Autodesk Fusion 360 part; units mm, degrees
(part 2 of 5)
sketch "Base" plane through (0, 0, 0) normal (0, 1, 0) x (1, 0, 0) in component "GM67 + printer"
  line L0 (0, 0) -> (183.0748, 0)
  line L1 (196.0652, -7.5) -> (240.6025, -84.641)
  line L2 (235.1122, -105.1314) -> (174.4904, -140.1314)
  line L3 (154, -134.641) -> (138.3301, -107.5)
  line L4 (125.3397, -100) -> (19, -100)
  line L5 (4, -115) -> (4, -142)
  line L6 (1, -145) -> (0, -145)
  line L7 (0, -145) -> (0, 0)
  arc A0 (196.0652, -7.5) -> (183.0748, 0) centre (183.0748, -15) ccw
  arc A1 (235.1122, -105.1314) -> (240.6025, -84.641) centre (227.6122, -92.141) ccw
  arc A2 (154, -134.641) -> (174.4904, -140.1314) centre (166.9904, -127.141) ccw
  arc A3 (138.3301, -107.5) -> (125.3397, -100) centre (125.3397, -115) ccw
  arc A4 (19, -100) -> (4, -115) centre (19, -115) ccw
  line L8 (4, -4) -> (183.0748, -4)
  arc A5 (192.6011, -9.5) -> (183.0748, -4) centre (183.0748, -15) ccw
  line L9 (192.6011, -9.5) -> (237.1384, -86.641)
  arc A6 (233.1122, -101.6673) -> (237.1384, -86.641) centre (227.6122, -92.141) ccw
  line L10 (233.1122, -101.6673) -> (172.4904, -136.6673)
  arc A7 (157.4641, -132.641) -> (172.4904, -136.6673) centre (166.9904, -127.141) ccw
  line L11 (157.4641, -132.641) -> (141.7942, -105.5)
  arc A8 (141.7942, -105.5) -> (125.3397, -96) centre (125.3397, -115) ccw
  line L12 (125.3397, -96) -> (19, -96)
  arc A9 (19, -96) -> (4, -103.3381) centre (19, -115) ccw
  line L13 (4, -103.3381) -> (4, -4)
  arc A10 (1, -145) -> (4, -142) centre (1, -142) ccw
  arc A11 (4, -12) -> (12, -4) centre (4, -4) ccw
  line L14 (4, -4) -> (9.6569, -9.6569) construction
  circle A12 centre (6.8284, -6.8284) radius 2
  line L15 (166.9904, -127.141) -> (161.5, -147.6314) construction
  spline S0 degree 2 poles (157.4641, -132.641) (166.9904, -127.141) (172.4904, -136.6673) knots 0 0 0 1.944544 1.944544 1.944544 weights 1 3 1
  circle A13 centre (165.1786, -133.9025) radius 2
  line L16 (192.6011, -9.5) -> (189.4806, -11.3016)
  line L17 (179.9994, -4) -> (179.9994, -6.8969)
  line L18 (181.9766, -9.7171) -> (186.9578, -11.5237)
  arc A14 (179.9994, -6.8969) -> (181.9766, -9.7171) centre (182.9994, -6.8969) ccw
  arc A15 (186.9578, -11.5237) -> (189.4806, -11.3016) centre (187.9806, -8.7035) ccw
  spline S1 degree 2 poles (233.1122, -101.6673) (227.6122, -92.141) (237.1384, -86.641) knots 0 0 0 1.944544 1.944544 1.944544 weights 1 3 1
  line L19 (227.6122, -92.141) -> (248.1025, -97.6314) construction
  circle A16 centre (234.3736, -93.9527) radius 2
  line L20 (179.9994, -4) -> (192.6011, -9.5) construction
  arc A17 (125.3397, -96) -> (109.3397, -96) centre (117.3397, -96) ccw
  line L21 (117.3397, -96) -> (117.3397, -88) construction
  circle A18 centre (117.3397, -93.1716) radius 2
  line L22 (4, -115) -> (0, -115)
  line L23 (186.3002, -6.75) -> (184.4672, -10.6204) construction
  circle A19 centre (185.872, -7.6542) radius 2
  circle A20 centre (6.8284, -6.8284) radius 2.25
  circle A21 centre (185.872, -7.6542) radius 2.25
  circle A22 centre (234.3736, -93.9527) radius 2.25
  circle A23 centre (117.3397, -93.1716) radius 2.25
  circle A24 centre (165.1786, -133.9025) radius 2.25
  line L24 (4, -53.669) -> (218.1021, -53.669) construction
  line L25 (135, -17.169) -> (72, -17.169)
  line L26 (72, -17.169) -> (72, -80.169)
  line L27 (72, -80.169) -> (135, -80.169)
  line L28 (135, -80.169) -> (135, -17.169)
  line L29 (135, -17.169) -> (72, -80.169) construction
  line L30 (72, -17.169) -> (135, -80.169) construction
  line L31 (133, -19.169) -> (74, -19.169)
  line L32 (74, -19.169) -> (74, -78.169) construction
  line L33 (74, -78.169) -> (133, -78.169) construction
  line L34 (133, -78.169) -> (133, -19.169) construction
  line L35 (133, -19.169) -> (74, -78.169) construction
  line L36 (74, -19.169) -> (133, -78.169) construction
  circle A25 centre (74, -78.169) radius 0.95
  circle A26 centre (74, -78.169) radius 3.45
  circle A27 centre (133, -78.169) radius 0.95
  circle A28 centre (133, -78.169) radius 3.45
  circle A29 centre (133, -19.169) radius 0.95
  circle A30 centre (133, -19.169) radius 3.45
  circle A31 centre (74, -19.169) radius 3.45
  circle A32 centre (74, -19.169) radius 0.95
  line L37 (49.5, -96) -> (49.5, -4)
  line L38 (53.5, -96) -> (53.5, -4)
  line L39 (53.5, -96) -> (53.5, -100)
  line L40 (53.5, -4) -> (53.5, 0)
  arc A33 (61.5, -96) -> (53.5, -88) centre (53.5, -96) ccw
  line L41 (53.5, -96) -> (59.1569, -90.3431) construction
  circle A34 centre (56.3284, -93.1716) radius 2
  circle A35 centre (56.3284, -93.1716) radius 2.25
  arc A36 (53.5, -12) -> (61.5, -4) centre (53.5, -4) ccw
  line L42 (53.5, -4) -> (59.1569, -9.6569) construction
  circle A37 centre (56.3284, -6.8284) radius 2
  circle A38 centre (56.3284, -6.8284) radius 2.25
  line L43 (49.5, -96) -> (4, -96)
  arc A39 (12, -96) -> (4, -88) centre (4, -96) ccw
  line L44 (4, -96) -> (9.6569, -90.3431) construction
  circle A40 centre (6.8284, -93.1716) radius 2
  circle A41 centre (6.8284, -93.1716) radius 2.25
  line L45 (117.3397, -96) -> (117.3397, -4) construction
  arc A42 (109.3397, -4) -> (125.3397, -4) centre (117.3397, -4) ccw
  line L46 (117.3397, -12) -> (117.3397, -4) construction
  line L47 (56.3284, -6.8284) -> (117.3397, -6.8284) construction
  circle A43 centre (117.3397, -6.8284) radius 2
  line L48 (56.3284, -93.1716) -> (117.3397, -93.1716) construction
  circle A44 centre (117.3397, -6.8284) radius 2.25
  line L49 (47.5, -96) -> (47.5, -95)
  line L50 (47.5, -95) -> (47.5, -4) construction
  line L51 (47.5, -12) -> (49.5, -12)
  arc A45 (47.5, -88) -> (39.5, -96) centre (47.5, -96) ccw
  line L52 (47.5, -88) -> (49.5, -88)
  line L53 (47.5, -96) -> (41.8431, -90.3431) construction
  circle A46 centre (44.6716, -93.1716) radius 2
  circle A47 centre (44.6716, -93.1716) radius 2.25
  arc A48 (39.5, -4) -> (47.5, -12) centre (47.5, -4) ccw
  line L54 (47.5, -4) -> (41.8431, -9.6569) construction
  circle A49 centre (44.6716, -6.8284) radius 2
  circle A50 centre (44.6716, -6.8284) radius 2.25
  line L55 (203.6221, -48.669) -> (205, -52.2911)
  line L56 (205, -52.2911) -> (204.352, -52.2911)
  line L57 (204.352, -52.2911) -> (203.5744, -50.122)
  spline S2 degree 2 poles (203.5744, -50.122) (203.4482, -49.7707) (203.3424, -49.3921) knots 0 0 0 1 1 1
  spline S3 degree 2 poles (203.3424, -49.3921) (203.2606, -49.6786) (203.1139, -50.0811) knots 0 0 0 1 1 1
  line L58 (203.1139, -50.0811) -> (202.309, -52.2911)
  line L59 (202.309, -52.2911) -> (201.678, -52.2911)
  line L60 (201.678, -52.2911) -> (203.0491, -48.669)
  line L61 (203.0491, -48.669) -> (203.6221, -48.669)
  spline S4 degree 2 poles (198.7722, -49.1158) (199.1132, -48.8259) (199.4287, -48.7066) knots 0 0 0 1 1 1
  spline S5 degree 2 poles (199.4287, -48.7066) (199.7442, -48.5872) (200.1057, -48.5872) knots 0 0 0 1 1 1
  spline S6 degree 2 poles (200.1057, -48.5872) (200.7026, -48.5872) (201.0232, -48.8788) knots 0 0 0 1 1 1
  spline S7 degree 2 poles (201.0232, -48.8788) (201.3438, -49.1704) (201.3438, -49.624) knots 0 0 0 1 1 1
  spline S8 degree 2 poles (201.3438, -49.624) (201.3438, -49.8901) (201.2227, -50.11) knots 0 0 0 1 1 1
  spline S9 degree 2 poles (201.2227, -50.11) (201.1016, -50.33) (200.9055, -50.463) knots 0 0 0 1 1 1
  spline S10 degree 2 poles (200.9055, -50.463) (200.7094, -50.5961) (200.4638, -50.6643) knots 0 0 0 1 1 1
  spline S11 degree 2 poles (200.4638, -50.6643) (200.2831, -50.712) (199.9181, -50.7564) knots 0 0 0 1 1 1
  spline S12 degree 2 poles (199.9181, -50.7564) (199.1746, -50.845) (198.8233, -50.9678) knots 0 0 0 1 1 1
  spline S13 degree 2 poles (198.8233, -50.9678) (198.8199, -51.094) (198.8199, -51.1281) knots 0 0 0 1 1 1
  spline S14 degree 2 poles (198.8199, -51.1281) (198.8199, -51.5033) (198.9939, -51.6568) knots 0 0 0 1 1 1
  spline S15 degree 2 poles (198.9939, -51.6568) (199.2292, -51.8648) (199.693, -51.8648) knots 0 0 0 1 1 1
  spline S16 degree 2 poles (199.693, -51.8648) (200.1262, -51.8648) (200.3325, -51.713) knots 0 0 0 1 1 1
  spline S17 degree 2 poles (200.3325, -51.713) (200.5389, -51.5613) (200.6378, -51.1759) knots 0 0 0 1 1 1
  line L62 (200.6378, -51.1759) -> (201.2381, -51.2577)
  spline S18 degree 2 poles (201.2381, -51.2577) (201.1562, -51.6431) (200.9686, -51.8802) knots 0 0 0 1 1 1
  spline S19 degree 2 poles (200.9686, -51.8802) (200.781, -52.1172) (200.4263, -52.2451) knots 0 0 0 1 1 1
  spline S20 degree 2 poles (200.4263, -52.2451) (200.0716, -52.373) (199.6044, -52.373) knots 0 0 0 1 1 1
  spline S21 degree 2 poles (199.6044, -52.373) (199.1405, -52.373) (198.8506, -52.2639) knots 0 0 0 1 1 1
  spline S22 degree 2 poles (198.8506, -52.2639) (198.5607, -52.1547) (198.4243, -51.9893) knots 0 0 0 1 1 1
  spline S23 degree 2 poles (198.4243, -51.9893) (198.2879, -51.8239) (198.2333, -51.5715) knots 0 0 0 1 1 1
  spline S24 degree 2 poles (198.2333, -51.5715) (198.2026, -51.4146) (198.2026, -51.0053) knots 0 0 0 1 1 1
  line L63 (198.2026, -51.0053) -> (198.2026, -50.1868)
  spline S25 degree 2 poles (198.2026, -50.1868) (198.2026, -49.3307) (198.1634, -49.1039) knots 0 0 0 1 1 1
  spline S26 degree 2 poles (198.1634, -49.1039) (198.1241, -48.8771) (198.0082, -48.669) knots 0 0 0 1 1 1
  line L64 (198.0082, -48.669) -> (198.6494, -48.669)
  spline S27 degree 2 poles (198.6494, -48.669) (198.7449, -48.86) (198.7722, -49.1158) knots 0 0 0 1 1 1
  spline S28 degree 2 poles (198.8233, -50.4869) (199.1576, -50.3505) (199.8261, -50.255) knots 0 0 0 1 1 1
  spline S29 degree 2 poles (199.8261, -50.255) (200.2046, -50.2004) (200.3615, -50.1322) knots 0 0 0 1 1 1
  spline S30 degree 2 poles (200.3615, -50.1322) (200.5184, -50.064) (200.6037, -49.9327) knots 0 0 0 1 1 1
  spline S31 degree 2 poles (200.6037, -49.9327) (200.6889, -49.8014) (200.6889, -49.6411) knots 0 0 0 1 1 1
  spline S32 degree 2 poles (200.6889, -49.6411) (200.6889, -49.3955) (200.5031, -49.2318) knots 0 0 0 1 1 1
  spline S33 degree 2 poles (200.5031, -49.2318) (200.3172, -49.0681) (199.9591, -49.0681) knots 0 0 0 1 1 1
  spline S34 degree 2 poles (199.9591, -49.0681) (199.6044, -49.0681) (199.3281, -49.2233) knots 0 0 0 1 1 1
  spline S35 degree 2 poles (199.3281, -49.2233) (199.0518, -49.3785) (198.9222, -49.6479) knots 0 0 0 1 1 1
  spline S36 degree 2 poles (198.9222, -49.6479) (198.8233, -49.856) (198.8233, -50.2618) knots 0 0 0 1 1 1
  line L65 (198.8233, -50.2618) -> (198.8233, -50.4869)
  line L66 (197.251, -48.669) -> (197.251, -52.2911)
  line L67 (197.251, -52.2911) -> (196.6985, -52.2911)
  line L68 (196.6985, -52.2911) -> (196.6985, -51.7761)
  spline S37 degree 2 poles (196.6985, -51.7761) (196.2995, -52.373) (195.5457, -52.373) knots 0 0 0 1 1 1
  spline S38 degree 2 poles (195.5457, -52.373) (195.2183, -52.373) (194.9437, -52.2553) knots 0 0 0 1 1 1
  spline S39 degree 2 poles (194.9437, -52.2553) (194.6692, -52.1377) (194.5327, -51.9467) knots 0 0 0 1 1 1
  spline S40 degree 2 poles (194.5327, -51.9467) (194.3963, -51.7557) (194.3417, -51.4931) knots 0 0 0 1 1 1
  spline S41 degree 2 poles (194.3417, -51.4931) (194.3076, -51.3225) (194.3076, -50.8962) knots 0 0 0 1 1 1
  line L69 (194.3076, -50.8962) -> (194.3076, -48.669)
  line L70 (194.3076, -48.669) -> (194.9216, -48.669)
  line L71 (194.9216, -48.669) -> (194.9216, -50.8723)
  spline S42 degree 2 poles (194.9216, -50.8723) (194.9216, -51.2475) (194.9932, -51.4334) knots 0 0 0 1 1 1
  spline S43 degree 2 poles (194.9932, -51.4334) (195.0648, -51.6193) (195.2473, -51.7301) knots 0 0 0 1 1 1
  spline S44 degree 2 poles (195.2473, -51.7301) (195.4297, -51.8409) (195.6753, -51.8409) knots 0 0 0 1 1 1
  spline S45 degree 2 poles (195.6753, -51.8409) (196.0675, -51.8409) (196.3523, -51.592) knots 0 0 0 1 1 1
  spline S46 degree 2 poles (196.3523, -51.592) (196.6371, -51.343) (196.6371, -50.6472) knots 0 0 0 1 1 1
  line L72 (196.6371, -50.6472) -> (196.6371, -48.669)
  line L73 (196.6371, -48.669) -> (197.251, -48.669)
  line L74 (191.3267, -48.669) -> (191.3267, -53.669)
  line L75 (191.3267, -53.669) -> (190.6651, -53.669)
  line L76 (190.6651, -53.669) -> (190.6651, -51.6158)
  line L77 (190.6651, -51.6158) -> (188.0662, -51.6158)
  line L78 (188.0662, -51.6158) -> (188.0662, -53.669)
  line L79 (188.0662, -53.669) -> (187.4045, -53.669)
  line L80 (187.4045, -53.669) -> (187.4045, -48.669)
  line L81 (187.4045, -48.669) -> (188.0662, -48.669)
  line L82 (188.0662, -48.669) -> (188.0662, -51.0258)
  line L83 (188.0662, -51.0258) -> (190.6651, -51.0258)
  line L84 (190.6651, -51.0258) -> (190.6651, -48.669)
  line L85 (190.6651, -48.669) -> (191.3267, -48.669)
  line L86 (183.9018, -49.8355) -> (183.2674, -49.757)
  spline S47 degree 2 poles (183.2674, -49.757) (183.4175, -49.2011) (183.8233, -48.8942) knots 0 0 0 1 1 1
  spline S48 degree 2 poles (183.8233, -48.8942) (184.2292, -48.5872) (184.8602, -48.5872) knots 0 0 0 1 1 1
  spline S49 degree 2 poles (184.8602, -48.5872) (185.6548, -48.5872) (186.1204, -49.0766) knots 0 0 0 1 1 1
  spline S50 degree 2 poles (186.1204, -49.0766) (186.5859, -49.566) (186.5859, -50.4494) knots 0 0 0 1 1 1
  spline S51 degree 2 poles (186.5859, -50.4494) (186.5859, -51.3635) (186.1153, -51.8682) knots 0 0 0 1 1 1
  spline S52 degree 2 poles (186.1153, -51.8682) (185.6446, -52.373) (184.8943, -52.373) knots 0 0 0 1 1 1
  spline S53 degree 2 poles (184.8943, -52.373) (184.1678, -52.373) (183.7074, -51.8785) knots 0 0 0 1 1 1
  spline S54 degree 2 poles (183.7074, -51.8785) (183.2469, -51.3839) (183.2469, -50.4869) knots 0 0 0 1 1 1
  spline S55 degree 2 poles (183.2469, -50.4869) (183.2469, -50.4323) (183.2503, -50.3232) knots 0 0 0 1 1 1
  line L87 (183.2503, -50.3232) -> (185.9516, -50.3232)
  spline S56 degree 2 poles (185.9516, -50.3232) (185.9175, -49.7263) (185.6139, -49.4092) knots 0 0 0 1 1 1
  spline S57 degree 2 poles (185.6139, -49.4092) (185.3104, -49.092) (184.8568, -49.092) knots 0 0 0 1 1 1
  spline S58 degree 2 poles (184.8568, -49.092) (184.5191, -49.092) (184.2804, -49.2693) knots 0 0 0 1 1 1
  spline S59 degree 2 poles (184.2804, -49.2693) (184.0416, -49.4467) (183.9018, -49.8355) knots 0 0 0 1 1 1
  line L88 (185.9175, -50.828) -> (183.895, -50.828)
  spline S60 degree 2 poles (183.895, -50.828) (183.9359, -51.285) (184.1269, -51.5135) knots 0 0 0 1 1 1
  spline S61 degree 2 poles (184.1269, -51.5135) (184.4202, -51.8682) (184.8874, -51.8682) knots 0 0 0 1 1 1
  spline S62 degree 2 poles (184.8874, -51.8682) (185.3104, -51.8682) (185.5986, -51.5851) knots 0 0 0 1 1 1
  spline S63 degree 2 poles (185.5986, -51.5851) (185.8868, -51.3021) (185.9175, -50.828) knots 0 0 0 1 1 1
  line L89 (182.4966, -48.669) -> (182.4966, -52.2911)
  line L90 (182.4966, -52.2911) -> (181.9475, -52.2911)
  line L91 (181.9475, -52.2911) -> (181.9475, -51.783)
  spline S64 degree 2 poles (181.9475, -51.783) (181.7769, -52.049) (181.4939, -52.211) knots 0 0 0 1 1 1
  spline S65 degree 2 poles (181.4939, -52.211) (181.2108, -52.373) (180.8493, -52.373) knots 0 0 0 1 1 1
  spline S66 degree 2 poles (180.8493, -52.373) (180.4468, -52.373) (180.1893, -52.2059) knots 0 0 0 1 1 1
  spline S67 degree 2 poles (180.1893, -52.2059) (179.9318, -52.0388) (179.8261, -51.7386) knots 0 0 0 1 1 1
  spline S68 degree 2 poles (179.8261, -51.7386) (179.3963, -52.373) (178.7074, -52.373) knots 0 0 0 1 1 1
  spline S69 degree 2 poles (178.7074, -52.373) (178.1685, -52.373) (177.8786, -52.0746) knots 0 0 0 1 1 1
  spline S70 degree 2 poles (177.8786, -52.0746) (177.5887, -51.7761) (177.5887, -51.1554) knots 0 0 0 1 1 1
  line L92 (177.5887, -51.1554) -> (177.5887, -48.669)
  line L93 (177.5887, -48.669) -> (178.1992, -48.669)
  line L94 (178.1992, -48.669) -> (178.1992, -50.9508)
  spline S71 degree 2 poles (178.1992, -50.9508) (178.1992, -51.3191) (178.2589, -51.4811) knots 0 0 0 1 1 1
  spline S72 degree 2 poles (178.2589, -51.4811) (178.3186, -51.6431) (178.4754, -51.742) knots 0 0 0 1 1 1
  spline S73 degree 2 poles (178.4754, -51.742) (178.6323, -51.8409) (178.8438, -51.8409) knots 0 0 0 1 1 1
  spline S74 degree 2 poles (178.8438, -51.8409) (179.2258, -51.8409) (179.4782, -51.5869) knots 0 0 0 1 1 1
  spline S75 degree 2 poles (179.4782, -51.5869) (179.7306, -51.3328) (179.7306, -50.7734) knots 0 0 0 1 1 1
  line L95 (179.7306, -50.7734) -> (179.7306, -48.669)
  line L96 (179.7306, -48.669) -> (180.3445, -48.669)
  line L97 (180.3445, -48.669) -> (180.3445, -51.0224)
  spline S76 degree 2 poles (180.3445, -51.0224) (180.3445, -51.4317) (180.4945, -51.6363) knots 0 0 0 1 1 1
  spline S77 degree 2 poles (180.4945, -51.6363) (180.6446, -51.8409) (180.9857, -51.8409) knots 0 0 0 1 1 1
  spline S78 degree 2 poles (180.9857, -51.8409) (181.2449, -51.8409) (181.4649, -51.7045) knots 0 0 0 1 1 1
  spline S79 degree 2 poles (181.4649, -51.7045) (181.6849, -51.5681) (181.7838, -51.3055) knots 0 0 0 1 1 1
  spline S80 degree 2 poles (181.7838, -51.3055) (181.8827, -51.0429) (181.8827, -50.5483) knots 0 0 0 1 1 1
  line L98 (181.8827, -50.5483) -> (181.8827, -48.669)
  line L99 (181.8827, -48.669) -> (182.4966, -48.669)
  line L100 (174.1985, -49.8355) -> (173.5641, -49.757)
  spline S81 degree 2 poles (173.5641, -49.757) (173.7142, -49.2011) (174.1201, -48.8942) knots 0 0 0 1 1 1
  spline S82 degree 2 poles (174.1201, -48.8942) (174.5259, -48.5872) (175.1569, -48.5872) knots 0 0 0 1 1 1
  spline S83 degree 2 poles (175.1569, -48.5872) (175.9516, -48.5872) (176.4171, -49.0766) knots 0 0 0 1 1 1
  spline S84 degree 2 poles (176.4171, -49.0766) (176.8827, -49.566) (176.8827, -50.4494) knots 0 0 0 1 1 1
  spline S85 degree 2 poles (176.8827, -50.4494) (176.8827, -51.3635) (176.412, -51.8682) knots 0 0 0 1 1 1
  spline S86 degree 2 poles (176.412, -51.8682) (175.9413, -52.373) (175.191, -52.373) knots 0 0 0 1 1 1
  spline S87 degree 2 poles (175.191, -52.373) (174.4645, -52.373) (174.0041, -51.8785) knots 0 0 0 1 1 1
  spline S88 degree 2 poles (174.0041, -51.8785) (173.5437, -51.3839) (173.5437, -50.4869) knots 0 0 0 1 1 1
  spline S89 degree 2 poles (173.5437, -50.4869) (173.5437, -50.4323) (173.5471, -50.3232) knots 0 0 0 1 1 1
  line L101 (173.5471, -50.3232) -> (176.2483, -50.3232)
  spline S90 degree 2 poles (176.2483, -50.3232) (176.2142, -49.7263) (175.9106, -49.4092) knots 0 0 0 1 1 1
  spline S91 degree 2 poles (175.9106, -49.4092) (175.6071, -49.092) (175.1535, -49.092) knots 0 0 0 1 1 1
  spline S92 degree 2 poles (175.1535, -49.092) (174.8158, -49.092) (174.5771, -49.2693) knots 0 0 0 1 1 1
  spline S93 degree 2 poles (174.5771, -49.2693) (174.3383, -49.4467) (174.1985, -49.8355) knots 0 0 0 1 1 1
  line L102 (176.2142, -50.828) -> (174.1917, -50.828)
  spline S94 degree 2 poles (174.1917, -50.828) (174.2326, -51.285) (174.4236, -51.5135) knots 0 0 0 1 1 1
  spline S95 degree 2 poles (174.4236, -51.5135) (174.7169, -51.8682) (175.1842, -51.8682) knots 0 0 0 1 1 1
  spline S96 degree 2 poles (175.1842, -51.8682) (175.6071, -51.8682) (175.8953, -51.5851) knots 0 0 0 1 1 1
  spline S97 degree 2 poles (175.8953, -51.5851) (176.1835, -51.3021) (176.2142, -50.828) knots 0 0 0 1 1 1
  line L103 (172.8001, -48.669) -> (172.8001, -52.2911)
  line L104 (172.8001, -52.2911) -> (172.2476, -52.2911)
  line L105 (172.2476, -52.2911) -> (172.2476, -51.742)
  spline S98 degree 2 poles (172.2476, -51.742) (172.0362, -52.1274) (171.8571, -52.2502) knots 0 0 0 1 1 1
  spline S99 degree 2 poles (171.8571, -52.2502) (171.678, -52.373) (171.4632, -52.373) knots 0 0 0 1 1 1
  spline S100 degree 2 poles (171.4632, -52.373) (171.1528, -52.373) (170.8322, -52.1752) knots 0 0 0 1 1 1
  line L106 (170.8322, -52.1752) -> (171.0437, -51.6056)
  spline S101 degree 2 poles (171.0437, -51.6056) (171.2688, -51.7386) (171.4939, -51.7386) knots 0 0 0 1 1 1
  spline S102 degree 2 poles (171.4939, -51.7386) (171.6951, -51.7386) (171.8554, -51.6175) knots 0 0 0 1 1 1
  spline S103 degree 2 poles (171.8554, -51.6175) (172.0157, -51.4965) (172.0839, -51.2816) knots 0 0 0 1 1 1
  spline S104 degree 2 poles (172.0839, -51.2816) (172.1862, -50.9542) (172.1862, -50.5654) knots 0 0 0 1 1 1
  line L107 (172.1862, -50.5654) -> (172.1862, -48.669)
  line L108 (172.1862, -48.669) -> (172.8001, -48.669)
  line L109 (169.1269, -49.2182) -> (169.0382, -48.6759)
  spline S105 degree 2 poles (169.0382, -48.6759) (169.2974, -48.6213) (169.502, -48.6213) knots 0 0 0 1 1 1
  spline S106 degree 2 poles (169.502, -48.6213) (169.8363, -48.6213) (170.0205, -48.727) knots 0 0 0 1 1 1
  spline S107 degree 2 poles (170.0205, -48.727) (170.2046, -48.8328) (170.2797, -49.005) knots 0 0 0 1 1 1
  spline S108 degree 2 poles (170.2797, -49.005) (170.3547, -49.1772) (170.3547, -49.7298) knots 0 0 0 1 1 1
  line L110 (170.3547, -49.7298) -> (170.3547, -51.8137)
  line L111 (170.3547, -51.8137) -> (170.8049, -51.8137)
  line L112 (170.8049, -51.8137) -> (170.8049, -52.2911)
  line L113 (170.8049, -52.2911) -> (170.3547, -52.2911)
  line L114 (170.3547, -52.2911) -> (170.3547, -53.1881)
  line L115 (170.3547, -53.1881) -> (169.7442, -53.5565)
  line L116 (169.7442, -53.5565) -> (169.7442, -52.2911)
  line L117 (169.7442, -52.2911) -> (169.1269, -52.2911)
  line L118 (169.1269, -52.2911) -> (169.1269, -51.8137)
  line L119 (169.1269, -51.8137) -> (169.7442, -51.8137)
  line L120 (169.7442, -51.8137) -> (169.7442, -49.6957)
  spline S109 degree 2 poles (169.7442, -49.6957) (169.7442, -49.433) (169.7118, -49.358) knots 0 0 0 1 1 1
  spline S110 degree 2 poles (169.7118, -49.358) (169.6794, -49.283) (169.6061, -49.2386) knots 0 0 0 1 1 1
  spline S111 degree 2 poles (169.6061, -49.2386) (169.5327, -49.1943) (169.3963, -49.1943) knots 0 0 0 1 1 1
  spline S112 degree 2 poles (169.3963, -49.1943) (169.294, -49.1943) (169.1269, -49.2182) knots 0 0 0 1 1 1
  line L121 (204.5293, -40.8655) -> (204.5293, -45.8655)
  line L122 (204.5293, -45.8655) -> (203.8677, -45.8655)
  line L123 (203.8677, -45.8655) -> (203.8677, -43.8123)
  line L124 (203.8677, -43.8123) -> (201.2688, -43.8123)
  line L125 (201.2688, -43.8123) -> (201.2688, -45.8655)
  line L126 (201.2688, -45.8655) -> (200.6071, -45.8655)
  line L127 (200.6071, -45.8655) -> (200.6071, -40.8655)
  line L128 (200.6071, -40.8655) -> (201.2688, -40.8655)
  line L129 (201.2688, -40.8655) -> (201.2688, -43.2223)
  line L130 (201.2688, -43.2223) -> (203.8677, -43.2223)
  line L131 (203.8677, -43.2223) -> (203.8677, -40.8655)
  line L132 (203.8677, -40.8655) -> (204.5293, -40.8655)
  spline S113 degree 2 poles (199.8124, -42.6766) (199.8124, -43.6827) (199.2531, -44.167) knots 0 0 0 1 1 1
  spline S114 degree 2 poles (199.2531, -44.167) (198.7858, -44.5695) (198.1139, -44.5695) knots 0 0 0 1 1 1
  spline S115 degree 2 poles (198.1139, -44.5695) (197.367, -44.5695) (196.8929, -44.08) knots 0 0 0 1 1 1
  spline S116 degree 2 poles (196.8929, -44.08) (196.4188, -43.5906) (196.4188, -42.7277) knots 0 0 0 1 1 1
  spline S117 degree 2 poles (196.4188, -42.7277) (196.4188, -42.0285) (196.6286, -41.6278) knots 0 0 0 1 1 1
  spline S118 degree 2 poles (196.6286, -41.6278) (196.8383, -41.227) (197.2391, -41.0053) knots 0 0 0 1 1 1
  spline S119 degree 2 poles (197.2391, -41.0053) (197.6398, -40.7836) (198.1139, -40.7836) knots 0 0 0 1 1 1
  spline S120 degree 2 poles (198.1139, -40.7836) (198.8745, -40.7836) (199.3435, -41.2714) knots 0 0 0 1 1 1
  spline S121 degree 2 poles (199.3435, -41.2714) (199.8124, -41.7591) (199.8124, -42.6766) knots 0 0 0 1 1 1
  spline S122 degree 2 poles (199.1814, -42.6766) (199.1814, -41.9808) (198.8779, -41.6346) knots 0 0 0 1 1 1
  spline S123 degree 2 poles (198.8779, -41.6346) (198.5744, -41.2884) (198.1139, -41.2884) knots 0 0 0 1 1 1
  spline S124 degree 2 poles (198.1139, -41.2884) (197.6569, -41.2884) (197.3533, -41.6363) knots 0 0 0 1 1 1
  spline S125 degree 2 poles (197.3533, -41.6363) (197.0498, -41.9842) (197.0498, -42.697) knots 0 0 0 1 1 1
  spline S126 degree 2 poles (197.0498, -42.697) (197.0498, -43.3689) (197.355, -43.7151) knots 0 0 0 1 1 1
  spline S127 degree 2 poles (197.355, -43.7151) (197.6603, -44.0613) (198.1139, -44.0613) knots 0 0 0 1 1 1
  spline S128 degree 2 poles (198.1139, -44.0613) (198.5744, -44.0613) (198.8779, -43.7168) knots 0 0 0 1 1 1
  spline S129 degree 2 poles (198.8779, -43.7168) (199.1814, -43.3723) (199.1814, -42.6766) knots 0 0 0 1 1 1
  line L133 (195.6992, -40.8655) -> (195.6992, -44.4876)
  line L134 (195.6992, -44.4876) -> (195.1501, -44.4876)
  line L135 (195.1501, -44.4876) -> (195.1501, -43.9794)
  spline S130 degree 2 poles (195.1501, -43.9794) (194.9795, -44.2454) (194.6965, -44.4075) knots 0 0 0 1 1 1
  spline S131 degree 2 poles (194.6965, -44.4075) (194.4134, -44.5695) (194.0518, -44.5695) knots 0 0 0 1 1 1
  spline S132 degree 2 poles (194.0518, -44.5695) (193.6494, -44.5695) (193.3919, -44.4023) knots 0 0 0 1 1 1
  spline S133 degree 2 poles (193.3919, -44.4023) (193.1344, -44.2352) (193.0286, -43.9351) knots 0 0 0 1 1 1
  spline S134 degree 2 poles (193.0286, -43.9351) (192.5989, -44.5695) (191.91, -44.5695) knots 0 0 0 1 1 1
  spline S135 degree 2 poles (191.91, -44.5695) (191.3711, -44.5695) (191.0812, -44.271) knots 0 0 0 1 1 1
  spline S136 degree 2 poles (191.0812, -44.271) (190.7913, -43.9726) (190.7913, -43.3519) knots 0 0 0 1 1 1
  line L136 (190.7913, -43.3519) -> (190.7913, -40.8655)
  line L137 (190.7913, -40.8655) -> (191.4018, -40.8655)
  line L138 (191.4018, -40.8655) -> (191.4018, -43.1472)
  spline S137 degree 2 poles (191.4018, -43.1472) (191.4018, -43.5156) (191.4615, -43.6776) knots 0 0 0 1 1 1
  spline S138 degree 2 poles (191.4615, -43.6776) (191.5211, -43.8396) (191.678, -43.9385) knots 0 0 0 1 1 1
  spline S139 degree 2 poles (191.678, -43.9385) (191.8349, -44.0374) (192.0464, -44.0374) knots 0 0 0 1 1 1
  spline S140 degree 2 poles (192.0464, -44.0374) (192.4284, -44.0374) (192.6808, -43.7833) knots 0 0 0 1 1 1
  spline S141 degree 2 poles (192.6808, -43.7833) (192.9332, -43.5292) (192.9332, -42.9699) knots 0 0 0 1 1 1
  line L139 (192.9332, -42.9699) -> (192.9332, -40.8655)
  line L140 (192.9332, -40.8655) -> (193.5471, -40.8655)
  line L141 (193.5471, -40.8655) -> (193.5471, -43.2188)
  spline S142 degree 2 poles (193.5471, -43.2188) (193.5471, -43.6281) (193.6971, -43.8328) knots 0 0 0 1 1 1
  spline S143 degree 2 poles (193.6971, -43.8328) (193.8472, -44.0374) (194.1883, -44.0374) knots 0 0 0 1 1 1
  spline S144 degree 2 poles (194.1883, -44.0374) (194.4475, -44.0374) (194.6675, -43.901) knots 0 0 0 1 1 1
  spline S145 degree 2 poles (194.6675, -43.901) (194.8874, -43.7645) (194.9864, -43.5019) knots 0 0 0 1 1 1
  spline S146 degree 2 poles (194.9864, -43.5019) (195.0853, -43.2393) (195.0853, -42.7448) knots 0 0 0 1 1 1
  line L142 (195.0853, -42.7448) -> (195.0853, -40.8655)
  line L143 (195.0853, -40.8655) -> (195.6992, -40.8655)
  line L144 (187.4011, -42.0319) -> (186.7667, -41.9535)
  spline S147 degree 2 poles (186.7667, -41.9535) (186.9168, -41.3976) (187.3226, -41.0906) knots 0 0 0 1 1 1
  spline S148 degree 2 poles (187.3226, -41.0906) (187.7285, -40.7836) (188.3595, -40.7836) knots 0 0 0 1 1 1
  spline S149 degree 2 poles (188.3595, -40.7836) (189.1542, -40.7836) (189.6197, -41.2731) knots 0 0 0 1 1 1
  spline S150 degree 2 poles (189.6197, -41.2731) (190.0853, -41.7625) (190.0853, -42.6459) knots 0 0 0 1 1 1
  spline S151 degree 2 poles (190.0853, -42.6459) (190.0853, -43.5599) (189.6146, -44.0647) knots 0 0 0 1 1 1
  spline S152 degree 2 poles (189.6146, -44.0647) (189.1439, -44.5695) (188.3936, -44.5695) knots 0 0 0 1 1 1
  spline S153 degree 2 poles (188.3936, -44.5695) (187.6671, -44.5695) (187.2067, -44.0749) knots 0 0 0 1 1 1
  spline S154 degree 2 poles (187.2067, -44.0749) (186.7462, -43.5804) (186.7462, -42.6834) knots 0 0 0 1 1 1
  spline S155 degree 2 poles (186.7462, -42.6834) (186.7462, -42.6288) (186.7497, -42.5197) knots 0 0 0 1 1 1
  line L145 (186.7497, -42.5197) -> (189.4509, -42.5197)
  spline S156 degree 2 poles (189.4509, -42.5197) (189.4168, -41.9228) (189.1132, -41.6056) knots 0 0 0 1 1 1
  spline S157 degree 2 poles (189.1132, -41.6056) (188.8097, -41.2884) (188.3561, -41.2884) knots 0 0 0 1 1 1
  spline S158 degree 2 poles (188.3561, -41.2884) (188.0184, -41.2884) (187.7797, -41.4658) knots 0 0 0 1 1 1
  spline S159 degree 2 poles (187.7797, -41.4658) (187.5409, -41.6431) (187.4011, -42.0319) knots 0 0 0 1 1 1
  line L146 (189.4168, -43.0244) -> (187.3943, -43.0244)
  spline S160 degree 2 poles (187.3943, -43.0244) (187.4352, -43.4815) (187.6262, -43.71) knots 0 0 0 1 1 1
  spline S161 degree 2 poles (187.6262, -43.71) (187.9195, -44.0647) (188.3868, -44.0647) knots 0 0 0 1 1 1
  spline S162 degree 2 poles (188.3868, -44.0647) (188.8097, -44.0647) (189.0979, -43.7816) knots 0 0 0 1 1 1
  spline S163 degree 2 poles (189.0979, -43.7816) (189.3861, -43.4985) (189.4168, -43.0244) knots 0 0 0 1 1 1
  line L147 (184.9113, -40.8655) -> (182.9911, -45.8655)
  line L148 (182.9911, -45.8655) -> (182.2783, -45.8655)
  line L149 (182.2783, -45.8655) -> (180.2319, -40.8655)
  line L150 (180.2319, -40.8655) -> (180.9857, -40.8655)
  line L151 (180.9857, -40.8655) -> (181.5689, -42.3798)
  line L152 (181.5689, -42.3798) -> (183.6596, -42.3798)
  line L153 (183.6596, -42.3798) -> (184.2087, -40.8655)
  line L154 (184.2087, -40.8655) -> (184.9113, -40.8655)
  line L155 (183.4686, -42.9187) -> (181.7735, -42.9187)
  line L156 (181.7735, -42.9187) -> (182.2954, -44.3034)
  spline S164 degree 2 poles (182.2954, -44.3034) (182.5341, -44.9344) (182.6501, -45.3403) knots 0 0 0 1 1 1
  spline S165 degree 2 poles (182.6501, -45.3403) (182.7456, -44.8594) (182.9195, -44.3853) knots 0 0 0 1 1 1
  line L157 (182.9195, -44.3853) -> (183.4686, -42.9187)
  line L158 (177.4079, -40.8655) -> (177.4079, -41.3976)
  spline S166 degree 2 poles (177.4079, -41.3976) (177.8308, -40.7836) (178.5573, -40.7836) knots 0 0 0 1 1 1
  spline S167 degree 2 poles (178.5573, -40.7836) (178.8779, -40.7836) (179.1559, -40.9064) knots 0 0 0 1 1 1
  spline S168 degree 2 poles (179.1559, -40.9064) (179.4338, -41.0292) (179.5686, -41.2151) knots 0 0 0 1 1 1
  spline S169 degree 2 poles (179.5686, -41.2151) (179.7033, -41.401) (179.7578, -41.6704) knots 0 0 0 1 1 1
  spline S170 degree 2 poles (179.7578, -41.6704) (179.7954, -41.8512) (179.7954, -42.2434) knots 0 0 0 1 1 1
  line L159 (179.7954, -42.2434) -> (179.7954, -44.4876)
  line L160 (179.7954, -44.4876) -> (179.1814, -44.4876)
  line L161 (179.1814, -44.4876) -> (179.1814, -42.4787)
  spline S171 degree 2 poles (179.1814, -42.4787) (179.1814, -41.9978) (179.1439, -41.8307) knots 0 0 0 1 1 1
  spline S172 degree 2 poles (179.1439, -41.8307) (179.0859, -41.5886) (178.8984, -41.4504) knots 0 0 0 1 1 1
  spline S173 degree 2 poles (178.8984, -41.4504) (178.7108, -41.3123) (178.4345, -41.3123) knots 0 0 0 1 1 1
  spline S174 degree 2 poles (178.4345, -41.3123) (178.1583, -41.3123) (177.9161, -41.4538) knots 0 0 0 1 1 1
  spline S175 degree 2 poles (177.9161, -41.4538) (177.6739, -41.5954) (177.5733, -41.8392) knots 0 0 0 1 1 1
  spline S176 degree 2 poles (177.5733, -41.8392) (177.4727, -42.0831) (177.4727, -42.5469) knots 0 0 0 1 1 1
  line L162 (177.4727, -42.5469) -> (177.4727, -44.4876)
  line L163 (177.4727, -44.4876) -> (176.8588, -44.4876)
  line L164 (176.8588, -44.4876) -> (176.8588, -40.8655)
  line L165 (176.8588, -40.8655) -> (177.4079, -40.8655)
  line L166 (174.5566, -41.4146) -> (174.4679, -40.8723)
  spline S177 degree 2 poles (174.4679, -40.8723) (174.7271, -40.8178) (174.9318, -40.8178) knots 0 0 0 1 1 1
  spline S178 degree 2 poles (174.9318, -40.8178) (175.266, -40.8178) (175.4502, -40.9235) knots 0 0 0 1 1 1
  spline S179 degree 2 poles (175.4502, -40.9235) (175.6344, -41.0292) (175.7094, -41.2014) knots 0 0 0 1 1 1
  spline S180 degree 2 poles (175.7094, -41.2014) (175.7844, -41.3737) (175.7844, -41.9262) knots 0 0 0 1 1 1
  line L167 (175.7844, -41.9262) -> (175.7844, -44.0101)
  line L168 (175.7844, -44.0101) -> (176.2347, -44.0101)
  line L169 (176.2347, -44.0101) -> (176.2347, -44.4876)
  line L170 (176.2347, -44.4876) -> (175.7844, -44.4876)
  line L171 (175.7844, -44.4876) -> (175.7844, -45.3846)
  line L172 (175.7844, -45.3846) -> (175.1739, -45.7529)
  line L173 (175.1739, -45.7529) -> (175.1739, -44.4876)
  line L174 (175.1739, -44.4876) -> (174.5566, -44.4876)
  line L175 (174.5566, -44.4876) -> (174.5566, -44.0101)
  line L176 (174.5566, -44.0101) -> (175.1739, -44.0101)
  line L177 (175.1739, -44.0101) -> (175.1739, -41.8921)
  spline S181 degree 2 poles (175.1739, -41.8921) (175.1739, -41.6295) (175.1415, -41.5545) knots 0 0 0 1 1 1
  spline S182 degree 2 poles (175.1415, -41.5545) (175.1091, -41.4794) (175.0358, -41.4351) knots 0 0 0 1 1 1
  spline S183 degree 2 poles (175.0358, -41.4351) (174.9625, -41.3907) (174.8261, -41.3907) knots 0 0 0 1 1 1
  spline S184 degree 2 poles (174.8261, -41.3907) (174.7237, -41.3907) (174.5566, -41.4146) knots 0 0 0 1 1 1
  spline S185 degree 2 poles (174.1849, -42.6766) (174.1849, -43.6827) (173.6255, -44.167) knots 0 0 0 1 1 1
  spline S186 degree 2 poles (173.6255, -44.167) (173.1583, -44.5695) (172.4864, -44.5695) knots 0 0 0 1 1 1
  spline S187 degree 2 poles (172.4864, -44.5695) (171.7394, -44.5695) (171.2653, -44.08) knots 0 0 0 1 1 1
  spline S188 degree 2 poles (171.2653, -44.08) (170.7913, -43.5906) (170.7913, -42.7277) knots 0 0 0 1 1 1
  spline S189 degree 2 poles (170.7913, -42.7277) (170.7913, -42.0285) (171.001, -41.6278) knots 0 0 0 1 1 1
  spline S190 degree 2 poles (171.001, -41.6278) (171.2108, -41.227) (171.6115, -41.0053) knots 0 0 0 1 1 1
  spline S191 degree 2 poles (171.6115, -41.0053) (172.0123, -40.7836) (172.4864, -40.7836) knots 0 0 0 1 1 1
  spline S192 degree 2 poles (172.4864, -40.7836) (173.2469, -40.7836) (173.7159, -41.2714) knots 0 0 0 1 1 1
  spline S193 degree 2 poles (173.7159, -41.2714) (174.1849, -41.7591) (174.1849, -42.6766) knots 0 0 0 1 1 1
  spline S194 degree 2 poles (173.5539, -42.6766) (173.5539, -41.9808) (173.2503, -41.6346) knots 0 0 0 1 1 1
  spline S195 degree 2 poles (173.2503, -41.6346) (172.9468, -41.2884) (172.4864, -41.2884) knots 0 0 0 1 1 1
  spline S196 degree 2 poles (172.4864, -41.2884) (172.0293, -41.2884) (171.7258, -41.6363) knots 0 0 0 1 1 1
  spline S197 degree 2 poles (171.7258, -41.6363) (171.4222, -41.9842) (171.4222, -42.697) knots 0 0 0 1 1 1
  spline S198 degree 2 poles (171.4222, -42.697) (171.4222, -43.3689) (171.7275, -43.7151) knots 0 0 0 1 1 1
  spline S199 degree 2 poles (171.7275, -43.7151) (172.0327, -44.0613) (172.4864, -44.0613) knots 0 0 0 1 1 1
  spline S200 degree 2 poles (172.4864, -44.0613) (172.9468, -44.0613) (173.2503, -43.7168) knots 0 0 0 1 1 1
  spline S201 degree 2 poles (173.2503, -43.7168) (173.5539, -43.3723) (173.5539, -42.6766) knots 0 0 0 1 1 1
  line L178 (170.0716, -40.8655) -> (170.0716, -44.4876)
  line L179 (170.0716, -44.4876) -> (169.5225, -44.4876)
  line L180 (169.5225, -44.4876) -> (169.5225, -43.9794)
  spline S202 degree 2 poles (169.5225, -43.9794) (169.352, -44.2454) (169.0689, -44.4075) knots 0 0 0 1 1 1
  spline S203 degree 2 poles (169.0689, -44.4075) (168.7858, -44.5695) (168.4243, -44.5695) knots 0 0 0 1 1 1
  spline S204 degree 2 poles (168.4243, -44.5695) (168.0218, -44.5695) (167.7643, -44.4023) knots 0 0 0 1 1 1
  spline S205 degree 2 poles (167.7643, -44.4023) (167.5068, -44.2352) (167.4011, -43.9351) knots 0 0 0 1 1 1
  spline S206 degree 2 poles (167.4011, -43.9351) (166.9713, -44.5695) (166.2824, -44.5695) knots 0 0 0 1 1 1
  spline S207 degree 2 poles (166.2824, -44.5695) (165.7435, -44.5695) (165.4536, -44.271) knots 0 0 0 1 1 1
  spline S208 degree 2 poles (165.4536, -44.271) (165.1637, -43.9726) (165.1637, -43.3519) knots 0 0 0 1 1 1
  line L181 (165.1637, -43.3519) -> (165.1637, -40.8655)
  line L182 (165.1637, -40.8655) -> (165.7742, -40.8655)
  line L183 (165.7742, -40.8655) -> (165.7742, -43.1472)
  spline S209 degree 2 poles (165.7742, -43.1472) (165.7742, -43.5156) (165.8339, -43.6776) knots 0 0 0 1 1 1
  spline S210 degree 2 poles (165.8339, -43.6776) (165.8936, -43.8396) (166.0505, -43.9385) knots 0 0 0 1 1 1
  spline S211 degree 2 poles (166.0505, -43.9385) (166.2074, -44.0374) (166.4188, -44.0374) knots 0 0 0 1 1 1
  spline S212 degree 2 poles (166.4188, -44.0374) (166.8008, -44.0374) (167.0532, -43.7833) knots 0 0 0 1 1 1
  spline S213 degree 2 poles (167.0532, -43.7833) (167.3056, -43.5292) (167.3056, -42.9699) knots 0 0 0 1 1 1
  line L184 (167.3056, -42.9699) -> (167.3056, -40.8655)
  line L185 (167.3056, -40.8655) -> (167.9195, -40.8655)
  line L186 (167.9195, -40.8655) -> (167.9195, -43.2188)
  spline S214 degree 2 poles (167.9195, -43.2188) (167.9195, -43.6281) (168.0696, -43.8328) knots 0 0 0 1 1 1
  spline S215 degree 2 poles (168.0696, -43.8328) (168.2196, -44.0374) (168.5607, -44.0374) knots 0 0 0 1 1 1
  spline S216 degree 2 poles (168.5607, -44.0374) (168.8199, -44.0374) (169.0399, -43.901) knots 0 0 0 1 1 1
  spline S217 degree 2 poles (169.0399, -43.901) (169.2599, -43.7645) (169.3588, -43.5019) knots 0 0 0 1 1 1
  spline S218 degree 2 poles (169.3588, -43.5019) (169.4577, -43.2393) (169.4577, -42.7448) knots 0 0 0 1 1 1
  line L187 (169.4577, -42.7448) -> (169.4577, -40.8655)
  line L188 (169.4577, -40.8655) -> (170.0716, -40.8655)
  spline S219 degree 2 poles (161.8895, -41.3123) (162.2306, -41.0224) (162.546, -40.903) knots 0 0 0 1 1 1
  spline S220 degree 2 poles (162.546, -40.903) (162.8615, -40.7836) (163.2231, -40.7836) knots 0 0 0 1 1 1
  spline S221 degree 2 poles (163.2231, -40.7836) (163.8199, -40.7836) (164.1405, -41.0753) knots 0 0 0 1 1 1
  spline S222 degree 2 poles (164.1405, -41.0753) (164.4611, -41.3669) (164.4611, -41.8205) knots 0 0 0 1 1 1
  spline S223 degree 2 poles (164.4611, -41.8205) (164.4611, -42.0865) (164.34, -42.3065) knots 0 0 0 1 1 1
  spline S224 degree 2 poles (164.34, -42.3065) (164.219, -42.5265) (164.0229, -42.6595) knots 0 0 0 1 1 1
  spline S225 degree 2 poles (164.0229, -42.6595) (163.8267, -42.7925) (163.5812, -42.8607) knots 0 0 0 1 1 1
  spline S226 degree 2 poles (163.5812, -42.8607) (163.4004, -42.9085) (163.0355, -42.9528) knots 0 0 0 1 1 1
  spline S227 degree 2 poles (163.0355, -42.9528) (162.292, -43.0415) (161.9407, -43.1643) knots 0 0 0 1 1 1
  spline S228 degree 2 poles (161.9407, -43.1643) (161.9372, -43.2905) (161.9372, -43.3246) knots 0 0 0 1 1 1
  spline S229 degree 2 poles (161.9372, -43.3246) (161.9372, -43.6997) (162.1112, -43.8532) knots 0 0 0 1 1 1
  spline S230 degree 2 poles (162.1112, -43.8532) (162.3465, -44.0613) (162.8104, -44.0613) knots 0 0 0 1 1 1
  spline S231 degree 2 poles (162.8104, -44.0613) (163.2435, -44.0613) (163.4499, -43.9095) knots 0 0 0 1 1 1
  spline S232 degree 2 poles (163.4499, -43.9095) (163.6562, -43.7577) (163.7551, -43.3723) knots 0 0 0 1 1 1
  line L189 (163.7551, -43.3723) -> (164.3554, -43.4542)
  spline S233 degree 2 poles (164.3554, -43.4542) (164.2735, -43.8396) (164.086, -44.0766) knots 0 0 0 1 1 1
  spline S234 degree 2 poles (164.086, -44.0766) (163.8984, -44.3137) (163.5437, -44.4416) knots 0 0 0 1 1 1
  spline S235 degree 2 poles (163.5437, -44.4416) (163.189, -44.5695) (162.7217, -44.5695) knots 0 0 0 1 1 1
  spline S236 degree 2 poles (162.7217, -44.5695) (162.2578, -44.5695) (161.9679, -44.4603) knots 0 0 0 1 1 1
  spline S237 degree 2 poles (161.9679, -44.4603) (161.678, -44.3512) (161.5416, -44.1858) knots 0 0 0 1 1 1
  spline S238 degree 2 poles (161.5416, -44.1858) (161.4052, -44.0203) (161.3506, -43.768) knots 0 0 0 1 1 1
  spline S239 degree 2 poles (161.3506, -43.768) (161.3199, -43.6111) (161.3199, -43.2018) knots 0 0 0 1 1 1
  line L190 (161.3199, -43.2018) -> (161.3199, -42.3832)
  spline S240 degree 2 poles (161.3199, -42.3832) (161.3199, -41.5272) (161.2807, -41.3004) knots 0 0 0 1 1 1
  spline S241 degree 2 poles (161.2807, -41.3004) (161.2415, -41.0736) (161.1255, -40.8655) knots 0 0 0 1 1 1
  line L191 (161.1255, -40.8655) -> (161.7667, -40.8655)
  spline S242 degree 2 poles (161.7667, -40.8655) (161.8622, -41.0565) (161.8895, -41.3123) knots 0 0 0 1 1 1
  spline S243 degree 2 poles (161.9407, -42.6834) (162.2749, -42.5469) (162.9434, -42.4514) knots 0 0 0 1 1 1
  spline S244 degree 2 poles (162.9434, -42.4514) (163.322, -42.3969) (163.4789, -42.3287) knots 0 0 0 1 1 1
  spline S245 degree 2 poles (163.4789, -42.3287) (163.6357, -42.2605) (163.721, -42.1291) knots 0 0 0 1 1 1
  spline S246 degree 2 poles (163.721, -42.1291) (163.8063, -41.9978) (163.8063, -41.8375) knots 0 0 0 1 1 1
  spline S247 degree 2 poles (163.8063, -41.8375) (163.8063, -41.592) (163.6204, -41.4283) knots 0 0 0 1 1 1
  spline S248 degree 2 poles (163.6204, -41.4283) (163.4345, -41.2645) (163.0764, -41.2645) knots 0 0 0 1 1 1
  spline S249 degree 2 poles (163.0764, -41.2645) (162.7217, -41.2645) (162.4454, -41.4197) knots 0 0 0 1 1 1
  spline S250 degree 2 poles (162.4454, -41.4197) (162.1692, -41.5749) (162.0396, -41.8444) knots 0 0 0 1 1 1
  spline S251 degree 2 poles (162.0396, -41.8444) (161.9407, -42.0524) (161.9407, -42.4583) knots 0 0 0 1 1 1
  line L192 (161.9407, -42.4583) -> (161.9407, -42.6834)
  line L193 (159.028, -41.4146) -> (158.9393, -40.8723)
  spline S252 degree 2 poles (158.9393, -40.8723) (159.1985, -40.8178) (159.4031, -40.8178) knots 0 0 0 1 1 1
  spline S253 degree 2 poles (159.4031, -40.8178) (159.7374, -40.8178) (159.9216, -40.9235) knots 0 0 0 1 1 1
  spline S254 degree 2 poles (159.9216, -40.9235) (160.1057, -41.0292) (160.1808, -41.2014) knots 0 0 0 1 1 1
  spline S255 degree 2 poles (160.1808, -41.2014) (160.2558, -41.3737) (160.2558, -41.9262) knots 0 0 0 1 1 1
  line L194 (160.2558, -41.9262) -> (160.2558, -44.0101)
  line L195 (160.2558, -44.0101) -> (160.706, -44.0101)
  line L196 (160.706, -44.0101) -> (160.706, -44.4876)
  line L197 (160.706, -44.4876) -> (160.2558, -44.4876)
  line L198 (160.2558, -44.4876) -> (160.2558, -45.3846)
  line L199 (160.2558, -45.3846) -> (159.6453, -45.7529)
  line L200 (159.6453, -45.7529) -> (159.6453, -44.4876)
  line L201 (159.6453, -44.4876) -> (159.028, -44.4876)
  line L202 (159.028, -44.4876) -> (159.028, -44.0101)
  line L203 (159.028, -44.0101) -> (159.6453, -44.0101)
  line L204 (159.6453, -44.0101) -> (159.6453, -41.8921)
  spline S256 degree 2 poles (159.6453, -41.8921) (159.6453, -41.6295) (159.6129, -41.5545) knots 0 0 0 1 1 1
  spline S257 degree 2 poles (159.6129, -41.5545) (159.5805, -41.4794) (159.5072, -41.4351) knots 0 0 0 1 1 1
  spline S258 degree 2 poles (159.5072, -41.4351) (159.4338, -41.3907) (159.2974, -41.3907) knots 0 0 0 1 1 1
  spline S259 degree 2 poles (159.2974, -41.3907) (159.1951, -41.3907) (159.028, -41.4146) knots 0 0 0 1 1 1
  line L205 (158.4243, -45.1595) -> (158.4243, -45.8655)
  line L206 (158.4243, -45.8655) -> (157.8104, -45.8655)
  line L207 (157.8104, -45.8655) -> (157.8104, -45.1595)
  line L208 (157.8104, -45.1595) -> (158.4243, -45.1595)
  line L209 (158.4243, -40.8655) -> (158.4243, -44.4876)
  line L210 (158.4243, -44.4876) -> (157.8104, -44.4876)
  line L211 (157.8104, -44.4876) -> (157.8104, -40.8655)
  line L212 (157.8104, -40.8655) -> (158.4243, -40.8655)
  spline S260 degree 2 poles (157.1044, -42.6766) (157.1044, -43.6827) (156.545, -44.167) knots 0 0 0 1 1 1
  spline S261 degree 2 poles (156.545, -44.167) (156.0778, -44.5695) (155.4059, -44.5695) knots 0 0 0 1 1 1
  spline S262 degree 2 poles (155.4059, -44.5695) (154.6589, -44.5695) (154.1849, -44.08) knots 0 0 0 1 1 1
  spline S263 degree 2 poles (154.1849, -44.08) (153.7108, -43.5906) (153.7108, -42.7277) knots 0 0 0 1 1 1
  spline S264 degree 2 poles (153.7108, -42.7277) (153.7108, -42.0285) (153.9205, -41.6278) knots 0 0 0 1 1 1
  spline S265 degree 2 poles (153.9205, -41.6278) (154.1303, -41.227) (154.531, -41.0053) knots 0 0 0 1 1 1
  spline S266 degree 2 poles (154.531, -41.0053) (154.9318, -40.7836) (155.4059, -40.7836) knots 0 0 0 1 1 1
  spline S267 degree 2 poles (155.4059, -40.7836) (156.1664, -40.7836) (156.6354, -41.2714) knots 0 0 0 1 1 1
  spline S268 degree 2 poles (156.6354, -41.2714) (157.1044, -41.7591) (157.1044, -42.6766) knots 0 0 0 1 1 1
  spline S269 degree 2 poles (156.4734, -42.6766) (156.4734, -41.9808) (156.1698, -41.6346) knots 0 0 0 1 1 1
  spline S270 degree 2 poles (156.1698, -41.6346) (155.8663, -41.2884) (155.4059, -41.2884) knots 0 0 0 1 1 1
  spline S271 degree 2 poles (155.4059, -41.2884) (154.9488, -41.2884) (154.6453, -41.6363) knots 0 0 0 1 1 1
  spline S272 degree 2 poles (154.6453, -41.6363) (154.3417, -41.9842) (154.3417, -42.697) knots 0 0 0 1 1 1
  spline S273 degree 2 poles (154.3417, -42.697) (154.3417, -43.3689) (154.647, -43.7151) knots 0 0 0 1 1 1
  spline S274 degree 2 poles (154.647, -43.7151) (154.9522, -44.0613) (155.4059, -44.0613) knots 0 0 0 1 1 1
  spline S275 degree 2 poles (155.4059, -44.0613) (155.8663, -44.0613) (156.1698, -43.7168) knots 0 0 0 1 1 1
  spline S276 degree 2 poles (156.1698, -43.7168) (156.4734, -43.3723) (156.4734, -42.6766) knots 0 0 0 1 1 1
  line L213 (152.9911, -40.8655) -> (152.9911, -44.4876)
  line L214 (152.9911, -44.4876) -> (152.4386, -44.4876)
  line L215 (152.4386, -44.4876) -> (152.4386, -43.9726)
  spline S277 degree 2 poles (152.4386, -43.9726) (152.0396, -44.5695) (151.2858, -44.5695) knots 0 0 0 1 1 1
  spline S278 degree 2 poles (151.2858, -44.5695) (150.9584, -44.5695) (150.6838, -44.4518) knots 0 0 0 1 1 1
  spline S279 degree 2 poles (150.6838, -44.4518) (150.4093, -44.3341) (150.2729, -44.1431) knots 0 0 0 1 1 1
  spline S280 degree 2 poles (150.2729, -44.1431) (150.1364, -43.9521) (150.0819, -43.6895) knots 0 0 0 1 1 1
  spline S281 degree 2 poles (150.0819, -43.6895) (150.0477, -43.519) (150.0477, -43.0927) knots 0 0 0 1 1 1
  line L216 (150.0477, -43.0927) -> (150.0477, -40.8655)
  line L217 (150.0477, -40.8655) -> (150.6617, -40.8655)
  line L218 (150.6617, -40.8655) -> (150.6617, -43.0688)
  spline S282 degree 2 poles (150.6617, -43.0688) (150.6617, -43.4439) (150.7333, -43.6298) knots 0 0 0 1 1 1
  spline S283 degree 2 poles (150.7333, -43.6298) (150.8049, -43.8157) (150.9874, -43.9266) knots 0 0 0 1 1 1
  spline S284 degree 2 poles (150.9874, -43.9266) (151.1698, -44.0374) (151.4154, -44.0374) knots 0 0 0 1 1 1
  spline S285 degree 2 poles (151.4154, -44.0374) (151.8076, -44.0374) (152.0924, -43.7884) knots 0 0 0 1 1 1
  spline S286 degree 2 poles (152.0924, -43.7884) (152.3772, -43.5394) (152.3772, -42.8437) knots 0 0 0 1 1 1
  line L219 (152.3772, -42.8437) -> (152.3772, -40.8655)
  line L220 (152.3772, -40.8655) -> (152.9911, -40.8655)
  point P0 (248.1025, -97.6314)
  point P1 (161.5, -147.6314)
  point P2 (134, -100)
  point P3 (4, -100)
  point P4 (4, -145)
  point P5 (188.2709, -12)
  point P6 (179.9994, -9)
  point P7 (103.5, -48.669)
  point P8 (103.5, -48.669)
  point P9 (103.5, -48.669)
  dimension "d1_2" = 130
  dimension "d2_2" = 100
  dimension "d3_2" = 100
  dimension "d4_2" = 55
  dimension "d5_2" = 4
  dimension "d7_2" = 45
  dimension "d8_2" = 120
  dimension "d9_2" = 4
  dimension "d40_2" = 15
  dimension "d47_2" = 3
  dimension "d84_3" = 8
  dimension "d85_2" = 4
  dimension "d88_2" = 19
  dimension "d94_2" = 15
  dimension "d95_2" = 19
  dimension "d96_2" = 15
  dimension "d101_2" = 11
  dimension "d102_2" = 15
  dimension "d105_2" = 7
  dimension "d111_2" = 5
  dimension "d112_2" = 5
  dimension "d113_2" = 3
  dimension "d115_2" = 7
  dimension "d120_2" = 8
  dimension "d121_2" = 8
  dimension "d139_2" = 1
  dimension "d147_2" = 0.25
  dimension "d148_2" = 0.25
  dimension "d149_2" = 0.25
  dimension "d150_2" = 0.25
  dimension "d153_2" = 3.2821
  dimension "d157_2" = 0.25
  dimension "d234_2" = 63
  dimension "d235_2" = 63
  dimension "d236_2" = 59
  dimension "d237_2" = 59
  dimension "d238_2" = 1.9
  dimension "d239_2" = 2.5
  dimension "d240_2" = 5
  dimension "d392" = 45.5
  dimension "d393" = 4
  dimension "d448" = 50
  dimension "d465" = 8
  dimension "d466" = 4
  dimension "d467" = 0.25
  dimension "d468" = 8
  dimension "d469" = 4
  dimension "d470" = 0.25
  dimension "d478" = 8
  dimension "d479" = 4
  dimension "d480" = 0.25
  dimension "d486" = 2.8284
  dimension "d487" = 2.8284
  dimension "d489" = 4
  dimension "d490" = 0.25
  dimension "d493" = 8
  dimension "d508" = 2
  dimension "d510" = 8
  dimension "d512" = 4
  dimension "d513" = 0.25
  dimension "d515" = 8
  dimension "d516" = 4
  dimension "d517" = 0.25
  constraint coincident L0.start L7.end
  constraint horizontal L0
  constraint perpendicular L1 L2
  constraint parallel L0 L4
  constraint perpendicular L4 L5
  constraint parallel L1 L3
  constraint perpendicular L5 L6
  constraint perpendicular L0 L7
  constraint tangent L0 A0
  constraint tangent L1 A0
  constraint coincident P0 L1
  constraint coincident P0 L2
  constraint tangent L1 A1
  constraint tangent L2 A1
  constraint equal A0 A1
  constraint coincident P1 L2
  constraint coincident P1 L3
  constraint tangent L2 A2
  constraint tangent L3 A2
  constraint equal A0 A2
  constraint coincident P2 L3
  constraint coincident P2 L4
  constraint tangent L3 A3
  constraint tangent L4 A3
  constraint equal A0 A3
  constraint coincident P3 L4
  constraint coincident P3 L5
  constraint tangent L4 A4
  constraint tangent L5 A4
  constraint equal A0 A4
  constraint coincident P4 L5
  constraint coincident P4 L6
  constraint tangent L5 A10
  constraint tangent L6 A10
  constraint coincident L13 A11.start
  constraint coincident L8 A11.end
  constraint coincident L8.start L13.end
  constraint midpoint A11 L14.end
  constraint midpoint L14 A12.centre
  constraint coincident A2.centre A7.centre
  constraint coincident P1 L15.end
  constraint coincident L15 A13.centre
  constraint equal A12 A13
  constraint perpendicular L9 L16
  constraint coincident L8 L17.start
  constraint perpendicular L8 L17
  constraint coincident P6 L17
  constraint coincident P6 L18
  constraint tangent L17 A14
  constraint tangent L18 A14
  constraint coincident P5 L18
  constraint coincident P5 L16
  constraint tangent L18 A15